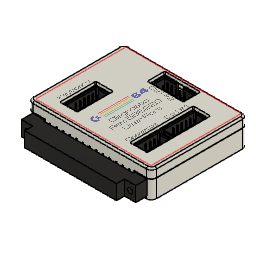
User_Port_Case_wHoles (Autodesk Fusion 360 design; units mm, degrees)
Autodesk Fusion 360 part; units mm, degrees
(part 1 of 2)
sketch "DXF import" plane through (0, 0, 0) normal (0, 0, 1) x (1, 0, 0) in component "PCB"
  arc A0 (0, 1) -> (1, 0) centre (1, 1) ccw
  line L0 (53, 1) -> (53, 54)
  line L1 (0, 1) -> (0, 54)
  arc A1 (53, 54) -> (52, 55) centre (52, 54) ccw
  line L2 (52, 55) -> (1, 55)
  line L3 (1, 0) -> (52, 0)
  arc A2 (1, 55) -> (0, 54) centre (1, 54) ccw
  arc A3 (52, 0) -> (53, 1) centre (52, 1) ccw
  line L4 (39.6875, 41.1163) -> (39.6875, 33.4963)
  line L5 (42.2275, 33.4963) -> (42.2275, 41.1163)
  line L6 (40.9575, 33.4963) -> (40.9575, 32.7343)
  line L7 (40.9575, 41.1163) -> (40.9575, 41.8783)
  line L8 (42.2275, 41.1163) -> (39.6875, 41.1163)
  line L9 (39.6875, 33.4963) -> (42.2275, 33.4963)
  line L10 (15.0813, 41.1163) -> (12.5412, 41.1163)
  line L11 (12.5412, 36.0363) -> (15.0813, 36.0363)
  line L12 (42.4713, 13.38) -> (39.9312, 13.38)
  line L13 (42.4713, 13.38) -> (42.4713, 8.3)
  line L14 (12.5412, 36.0363) -> (12.5412, 41.1163)
  line L15 (15.0813, 41.1163) -> (15.0813, 36.0363)
  line L16 (7.3025, 33.02) -> (12.3825, 33.02)
  line L17 (14.7637, 18.2563) -> (12.2238, 18.2563)
  line L18 (39.9312, 8.3) -> (42.4713, 8.3)
  line L19 (39.9312, 8.3) -> (39.9312, 13.38)
  circle A4 centre (4, 51) radius 3.1
  line L20 (32.6707, 40.7035) -> (32.6707, 34.8615)
  arc A5 (15.9068, 26.1303) -> (15.9068, 28.1623) centre (15.9068, 27.1463) ccw
  line L21 (15.9068, 30.0673) -> (15.9068, 28.1623)
  line L22 (15.9068, 34.8615) -> (32.6707, 34.8615)
  line L23 (15.9068, 24.2253) -> (15.9068, 26.1303)
  line L24 (12.2238, 13.1763) -> (12.2238, 18.2563)
  line L25 (15.9068, 24.2253) -> (32.6707, 24.2253)
  line L26 (32.6707, 30.0673) -> (32.6707, 24.2253)
  line L27 (32.6707, 30.0673) -> (15.9068, 30.0673)
  line L28 (50.18, 0) -> (50.18, -1)
  line L29 (32.6707, 40.7035) -> (15.9068, 40.7035)
  circle A6 centre (49, 51) radius 3.1
  line L30 (15.9068, 18.161) -> (15.9068, 16.256)
  line L31 (46.72, -1) -> (46.72, 0)
  line L32 (12.3825, 30.48) -> (12.3825, 33.02)
  line L33 (15.9068, 12.319) -> (15.9068, 14.224)
  circle A7 centre (49, 51) radius 1.5875
  line L34 (46.72, 0) -> (46.22, 0)
  line L35 (32.6707, 18.161) -> (15.9068, 18.161)
  arc A8 (15.9068, 14.224) -> (15.9068, 16.256) centre (15.9068, 15.24) ccw
  line L36 (15.9068, 12.319) -> (32.6707, 12.319)
  line L37 (32.6707, 18.161) -> (32.6707, 12.319)
  line L38 (49.45, 0.1) -> (49.45, -1)
  line L39 (47.45, 0.1) -> (47.45, -1)
  line L40 (46.22, 0) -> (46.22, -1)
  line L41 (50.68, -1) -> (50.68, 0)
  arc A9 (15.9068, 36.7665) -> (15.9068, 38.7985) centre (15.9068, 37.7825) ccw
  line L42 (50.68, 0) -> (50.18, 0)
  line L43 (31.61, 0.1) -> (31.61, -1)
  line L44 (15.9068, 40.7035) -> (15.9068, 38.7985)
  line L45 (12.2238, 13.1763) -> (14.7637, 13.1763)
  line L46 (14.7637, 18.2563) -> (14.7637, 13.1763)
  line L47 (12.3825, 30.48) -> (7.3025, 30.48)
  line L48 (7.3025, 33.02) -> (7.3025, 30.48)
  circle A10 centre (4, 51) radius 1.5875
  line L49 (15.9068, 34.8615) -> (15.9068, 36.7665)
  line L50 (22.96, 0) -> (22.46, 0)
  line L51 (7.85, 0.1) -> (7.85, -1)
  line L52 (42.76, -1) -> (42.76, 0)
  line L53 (43.49, 0.1) -> (43.49, -1)
  line L54 (45.49, 0.1) -> (45.49, -1)
  line L55 (30.88, -1) -> (30.88, 0)
  line L56 (7.12, -1) -> (7.12, 0)
  line L57 (22.46, 0) -> (22.46, -1)
  line L58 (7.12, 0) -> (6.62, 0)
  line L59 (35.57, 0.1) -> (35.57, -1)
  line L60 (6.62, 0) -> (6.62, -1)
  line L61 (14.54, 0) -> (14.54, -1)
  line L62 (37.57, 0.1) -> (37.57, -1)
  line L63 (38.8, -1) -> (38.8, 0)
  line L64 (15.04, 0) -> (14.54, 0)
  line L65 (18.5, 0) -> (18.5, -1)
  line L66 (29.65, 0.1) -> (29.65, -1)
  line L67 (30.88, 0) -> (30.38, 0)
  line L68 (27.65, 0.1) -> (27.65, -1)
  line L69 (26.42, 0) -> (26.42, -1)
  line L70 (38.8, 0) -> (38.3, 0)
  line L71 (34.84, 0) -> (34.34, 0)
  line L72 (39.53, 0.1) -> (39.53, -1)
  line L73 (42.26, 0) -> (42.26, -1)
  line L74 (42.76, 0) -> (42.26, 0)
  line L75 (26.92, -1) -> (26.92, 0)
  line L76 (38.3, 0) -> (38.3, -1)
  line L77 (33.61, 0.1) -> (33.61, -1)
  line L78 (34.34, 0) -> (34.34, -1)
  line L79 (26.92, 0) -> (26.42, 0)
  line L80 (30.38, 0) -> (30.38, -1)
  line L81 (34.84, -1) -> (34.84, 0)
  line L82 (41.53, 0.1) -> (41.53, -1)
  line L83 (21.73, 0.1) -> (21.73, -1)
  line L84 (15.77, 0.1) -> (15.77, -1)
  line L85 (11.08, -1) -> (11.08, 0)
  line L86 (23.69, 0.1) -> (23.69, -1)
  line L87 (19.73, 0.1) -> (19.73, -1)
  line L88 (25.69, 0.1) -> (25.69, -1)
  line L89 (19, -1) -> (19, 0)
  line L90 (11.81, 0.1) -> (11.81, -1)
  line L91 (54.17, -6.8) -> (54.17, -11.6)
  line L92 (11.08, 0) -> (10.58, 0)
  line L93 (22.96, -1) -> (22.96, 0)
  line L94 (55.97, -6.8) -> (54.17, -6.8)
  line L95 (-6.03, -6.8) -> (-7.58, -6.8)
  line L96 (59.37, -6.8) -> (55.97, -6.8)
  line L97 (60.92, -6.8) -> (59.37, -6.8)
  line L98 (19, 0) -> (18.5, 0)
  line L99 (9.85, 0.1) -> (9.85, -1)
  line L100 (53.47, 0) -> (53.47, -1)
  line L101 (3.16, -1) -> (3.16, 0)
  line L102 (17.77, 0.1) -> (17.77, -1)
  line L103 (-2.63, -6.8) -> (-2.63, -5.2)
  line L104 (-4.33, 0) -> (-4.33, -2.8667)
  line L105 (57.67, -3.6853) -> (57.67, -3.548)
  line L106 (55.97, -4.2) -> (55.97, -2.6)
  line L107 (59.37, -1.6) -> (59.37, 0)
  line L108 (60.92, 0) -> (59.37, 0)
  line L109 (59.37, 0) -> (57.67, 0)
  line L110 (-4.33, -3.548) -> (-4.33, -3.6853)
  line L111 (-4.33, -4.3667) -> (-4.33, -7.2333)
  line L112 (55.97, -1.6) -> (55.97, 0)
  line L113 (57.67, 0) -> (55.97, 0)
  line L114 (-0.83, -6.8) -> (-2.63, -6.8)
  line L115 (-2.63, -4.2) -> (-2.63, -2.6)
  line L116 (-4.33, -8.7333) -> (-4.33, -11.6)
  line L117 (-4.33, 0) -> (-6.03, 0)
  line L118 (10.58, 0) -> (10.58, -1)
  line L119 (13.81, 0.1) -> (13.81, -1)
  line L120 (5.89, 0.1) -> (5.89, -1)
  line L121 (-2.63, -1.6) -> (-2.63, 0)
  line L122 (-6.03, -1.6) -> (-6.03, 0)
  line L123 (55.97, 0) -> (53.47, 0)
  line L124 (-7.58, 0) -> (-7.58, -6.8)
  line L125 (3.16, 0) -> (2.66, 0)
  line L126 (3.89, 0.1) -> (3.89, -1)
  line L127 (15.04, -1) -> (15.04, 0)
  line L128 (59.37, -4.2) -> (59.37, -2.6)
  line L129 (-6.03, -6.8) -> (-6.03, -5.2)
  line L130 (2.66, 0) -> (2.66, -1)
  line L131 (51.81, 14.73) -> (52.6038, 14.73)
  line L132 (52.6038, 23.62) -> (52.6038, 17.27)
  line L133 (-0.13, 0) -> (-2.63, 0)
  line L134 (60.92, 0) -> (60.92, -6.8)
  line L135 (46.2537, 8.38) -> (44.825, 8.38)
  line L136 (51.81, 17.27) -> (52.6038, 17.27)
  line L137 (-0.83, -11.6) -> (-0.83, -6.8)
  line L138 (-6.03, 0) -> (-7.58, 0)
  line L139 (57.67, -2.8667) -> (57.67, 0)
  line L140 (51.3338, 17.27) -> (51.81, 17.27)
  line L141 (46.2537, 23.62) -> (52.6038, 23.62)
  line L142 (44.6662, 22.35) -> (44.825, 22.35)
  line L143 (51.3338, 9.65) -> (46.2537, 9.65)
  line L144 (44.825, 22.35) -> (44.825, 22.8263)
  line L145 (57.67, -11.6) -> (57.67, -8.7333)
  line L146 (43.3962, 23.62) -> (44.825, 23.62)
  line L147 (51.81, 14.73) -> (51.81, 9.1737)
  line L148 (46.2537, 22.35) -> (46.2537, 22.8263)
  line L149 (57.67, -7.2333) -> (57.67, -4.3667)
  line L150 (44.825, 8.38) -> (43.3962, 8.38)
  line L151 (51.3338, 22.35) -> (51.3338, 17.27)
  line L152 (44.825, 9.65) -> (44.825, 9.1737)
  line L153 (55.97, -6.8) -> (55.97, -5.2)
  line L154 (51.3338, 22.35) -> (51.81, 22.8263)
  line L155 (51.3338, 14.73) -> (51.3338, 9.65)
  line L156 (-4.33, -7.9147) -> (-4.33, -8.052)
  line L157 (53.47, -1) -> (-0.13, -1)
  line L158 (-2.63, -6.8) -> (-6.03, -6.8)
  line L159 (44.6662, 9.65) -> (44.6662, 22.35)
  line L160 (46.2537, 22.35) -> (51.3338, 22.35)
  line L161 (54.17, -11.6) -> (-0.83, -11.6)
  line L162 (57.67, -8.052) -> (57.67, -7.9147)
  line L163 (52.6038, 14.73) -> (52.6038, 8.38)
  line L164 (51.3338, 17.27) -> (51.3338, 14.73)
  line L165 (43.3962, 8.38) -> (43.3962, 23.62)
  line L166 (46.2537, 9.65) -> (44.825, 9.65)
  line L167 (51.3338, 14.73) -> (51.81, 14.73)
  line L168 (-6.03, -4.2) -> (-6.03, -2.6)
  line L169 (52.6038, 17.27) -> (52.6038, 14.73)
  line L170 (52.6038, 8.38) -> (46.2537, 8.38)
  line L171 (44.825, 9.65) -> (44.6662, 9.65)
  line L172 (59.37, -6.8) -> (59.37, -5.2)
  line L173 (44.825, 23.62) -> (46.2537, 23.62)
  line L174 (44.825, 22.35) -> (46.2537, 22.35)
  line L175 (-2.63, 0) -> (-4.33, 0)
  line L176 (-0.13, -1) -> (-0.13, 0)
  arc A11 (43.3962, 35.4763) -> (43.3962, 34.3651) centre (43.3962, 34.9207) ccw
  line L177 (46.2537, 9.1737) -> (51.81, 9.1737)
  line L178 (44.19, 9.1737) -> (44.6662, 9.65)
  arc A12 (43.3962, 10.92) -> (43.3962, 9.65) centre (43.3962, 10.285) ccw
  line L179 (44.825, 22.8263) -> (44.19, 22.8263)
  arc A13 (43.3962, 27.38) -> (43.3962, 26.11) centre (43.3962, 26.745) ccw
  line L180 (44.825, 24.84) -> (43.3962, 24.84)
  line L181 (44.825, 25.6337) -> (44.825, 24.84)
  line L182 (51.81, 25.6337) -> (51.3338, 26.11)
  arc A14 (43.3962, 22.35) -> (43.3962, 21.08) centre (43.3962, 21.715) ccw
  line L183 (44.19, 25.6337) -> (44.825, 25.6337)
  line L184 (44.6662, 26.11) -> (44.6662, 43.89)
  line L185 (44.825, 26.11) -> (44.6662, 26.11)
  line L186 (43.3962, 45.16) -> (44.825, 45.16)
  line L187 (46.2537, 44.3663) -> (46.2537, 45.16)
  line L188 (44.825, 43.89) -> (44.825, 44.3663)
  line L189 (51.81, 9.1737) -> (51.3338, 9.65)
  arc A15 (43.3962, 16.4763) -> (43.3962, 15.3651) centre (43.3962, 15.9207) ccw
  line L190 (46.2537, 22.8263) -> (46.2537, 23.62)
  line L191 (44.19, 9.1737) -> (44.825, 9.1737)
  line L192 (44.825, 9.1737) -> (44.825, 8.38)
  line L193 (51.81, 17.27) -> (51.81, 22.8263)
  line L194 (46.2537, 9.65) -> (46.2537, 9.1737)
  line L195 (46.2537, 22.8263) -> (51.81, 22.8263)
  line L196 (44.6662, 22.35) -> (44.19, 22.8263)
  line L197 (51.3338, 37.0638) -> (51.3338, 32.9362)
  line L198 (51.3338, 37.0638) -> (51.81, 37.0638)
  line L199 (44.825, 44.3663) -> (44.19, 44.3663)
  line L200 (51.3338, 43.89) -> (51.81, 44.3663)
  line L201 (44.825, 43.89) -> (46.2537, 43.89)
  line L202 (46.2537, 25.6337) -> (46.2537, 24.84)
  line L203 (51.3338, 43.89) -> (51.3338, 37.0638)
  line L204 (46.2537, 43.89) -> (46.2537, 44.3663)
  line L205 (51.81, 32.9362) -> (52.6038, 32.9362)
  line L206 (51.3338, 26.11) -> (46.2537, 26.11)
  line L207 (46.2537, 9.1737) -> (46.2537, 8.38)
  line L208 (44.19, 25.6337) -> (44.19, 44.3663)
  line L209 (44.19, 9.1737) -> (44.19, 22.8263)
  line L210 (46.2537, 25.6337) -> (51.81, 25.6337)
  line L211 (44.19, 25.6337) -> (44.6662, 26.11)
  line L212 (44.825, 22.8263) -> (44.825, 23.62)
  line L213 (51.81, 32.9362) -> (51.81, 25.6337)
  line L214 (44.6662, 43.89) -> (44.825, 43.89)
  arc A16 (43.3962, 43.89) -> (43.3962, 42.62) centre (43.3962, 43.255) ccw
  line L215 (44.825, 26.11) -> (44.825, 25.6337)
  line L216 (52.6038, 37.0638) -> (52.6038, 32.9362)
  line L217 (43.3962, 24.84) -> (43.3962, 45.16)
  line L218 (46.2537, 26.11) -> (44.825, 26.11)
  line L219 (44.825, 44.3663) -> (44.825, 45.16)
  line L220 (37.16, 46.825) -> (37.16, 45.3962)
  line L221 (18.11, 48.2537) -> (17.6337, 48.2537)
  line L222 (37.16, 54.6038) -> (37.16, 48.2537)
  arc A17 (26.5238, 45.3962) -> (27.635, 45.3962) centre (27.0794, 45.3962) ccw
  line L223 (51.3338, 32.9362) -> (51.3338, 26.11)
  line L224 (36.3663, 46.19) -> (36.3663, 46.825)
  line L225 (51.81, 37.0638) -> (51.81, 44.3663)
  line L226 (29.0638, 53.81) -> (29.0638, 54.6038)
  line L227 (29.0638, 53.3338) -> (35.89, 53.3338)
  line L228 (46.2537, 45.16) -> (52.6038, 45.16)
  line L229 (17.6337, 46.825) -> (16.84, 46.825)
  line L230 (37.16, 48.2537) -> (37.16, 46.825)
  line L231 (46.2537, 43.89) -> (51.3338, 43.89)
  line L232 (52.6038, 32.9362) -> (52.6038, 24.84)
  line L233 (18.11, 53.3338) -> (24.9362, 53.3338)
  line L234 (36.3663, 48.2537) -> (36.3663, 53.81)
  line L235 (52.6038, 45.16) -> (52.6038, 37.0638)
  line L236 (51.3338, 32.9362) -> (51.81, 32.9362)
  line L237 (44.6662, 43.89) -> (44.19, 44.3663)
  line L238 (17.6337, 46.825) -> (17.6337, 46.19)
  line L239 (18.11, 46.6662) -> (18.11, 46.825)
  line L240 (52.6038, 24.84) -> (46.2537, 24.84)
  line L241 (18.11, 46.825) -> (18.11, 48.2537)
  line L242 (24.9362, 53.81) -> (24.9362, 54.6038)
  line L243 (29.0638, 54.6038) -> (37.16, 54.6038)
  line L244 (29.0638, 53.3338) -> (29.0638, 53.81)
  line L245 (18.11, 46.825) -> (17.6337, 46.825)
  line L246 (36.3663, 46.19) -> (17.6337, 46.19)
  line L247 (46.2537, 44.3663) -> (51.81, 44.3663)
  line L248 (29.0638, 53.81) -> (36.3663, 53.81)
  line L249 (18.11, 53.3338) -> (17.6337, 53.81)
  line L250 (44.825, 45.16) -> (46.2537, 45.16)
  line L251 (46.2537, 24.84) -> (44.825, 24.84)
  arc A18 (18.11, 45.3962) -> (19.38, 45.3962) centre (18.745, 45.3962) ccw
  line L252 (24.9362, 53.3338) -> (29.0638, 53.3338)
  line L253 (46.2537, 26.11) -> (46.2537, 25.6337)
  line L254 (18.11, 46.6662) -> (17.6337, 46.19)
  line L255 (36.3663, 46.19) -> (35.89, 46.6662)
  line L256 (51.81, 37.0638) -> (52.6038, 37.0638)
  line L257 (35.89, 48.2537) -> (35.89, 46.825)
  line L258 (2.6987, 27.4638) -> (2.8575, 27.4638)
  line L259 (16.84, 46.825) -> (16.84, 48.2537)
  line L260 (9.3663, 9.6837) -> (4.2862, 9.6837)
  line L261 (9.8425, 20.6376) -> (9.8425, 27.9401)
  line L262 (18.11, 48.2537) -> (18.11, 53.3338)
  line L263 (4.2862, 28.7338) -> (10.6363, 28.7338)
  line L264 (9.3663, 16.5099) -> (9.3663, 9.6837)
  arc A19 (1.4287, 27.4638) -> (1.4287, 26.1938) centre (1.4287, 26.8288) ccw
  line L265 (10.6363, 28.7338) -> (10.6363, 20.6376)
  line L266 (2.8575, 9.6837) -> (2.6987, 9.6837)
  line L267 (24.9362, 53.3338) -> (24.9362, 53.81)
  arc A20 (34.62, 45.3962) -> (35.89, 45.3962) centre (35.255, 45.3962) ccw
  line L268 (9.3663, 20.6376) -> (9.3663, 16.5099)
  line L269 (17.6337, 48.2537) -> (16.84, 48.2537)
  line L270 (24.9362, 53.81) -> (17.6337, 53.81)
  line L271 (2.6987, 27.4638) -> (2.2225, 27.9401)
  line L272 (4.2862, 9.6837) -> (4.2862, 9.2074)
  line L273 (36.3663, 46.825) -> (37.16, 46.825)
  line L274 (16.84, 54.6038) -> (24.9362, 54.6038)
  line L275 (35.89, 48.2537) -> (36.3663, 48.2537)
  line L276 (17.6337, 48.2537) -> (17.6337, 53.81)
  line L277 (16.84, 45.3962) -> (16.84, 46.825)
  line L278 (35.89, 53.3338) -> (35.89, 48.2537)
  line L279 (10.6363, 20.6376) -> (10.6363, 16.5099)
  line L280 (2.8575, 28.7338) -> (4.2862, 28.7338)
  line L281 (35.89, 46.6662) -> (18.11, 46.6662)
  line L282 (24.9362, 54.6038) -> (29.0638, 54.6038)
  line L283 (1.4287, 28.7338) -> (2.8575, 28.7338)
  line L284 (35.89, 46.825) -> (36.3663, 46.825)
  line L285 (36.3663, 48.2537) -> (37.16, 48.2537)
  line L286 (35.89, 46.825) -> (35.89, 46.6662)
  line L287 (2.8575, 8.4138) -> (1.4287, 8.4138)
  line L288 (1.4287, 8.4138) -> (1.4287, 28.7338)
  line L289 (37.16, 45.3962) -> (16.84, 45.3962)
  line L290 (10.6363, 16.5099) -> (10.6363, 8.4138)
  line L291 (4.2862, 27.9401) -> (4.2862, 28.7338)
  arc A21 (1.4287, 10.9537) -> (1.4287, 9.6837) centre (1.4287, 10.3187) ccw
  line L292 (9.3663, 20.6376) -> (9.8425, 20.6376)
  line L293 (36.3663, 53.81) -> (35.89, 53.3338)
  line L294 (2.8575, 27.9401) -> (2.2225, 27.9401)
  line L295 (9.3663, 16.5099) -> (9.8425, 16.5099)
  line L296 (2.8575, 9.6837) -> (2.8575, 9.2074)
  line L297 (2.2225, 9.2074) -> (2.6987, 9.6837)
  arc A22 (1.4287, 19.05) -> (1.4287, 17.9388) centre (1.4287, 18.4944) ccw
  line L298 (16.84, 48.2537) -> (16.84, 54.6038)
  line L299 (4.2862, 27.4638) -> (9.3663, 27.4638)
  line L300 (36.6713, 26.035) -> (34.1313, 26.035)
  line L301 (38.1, 33.4963) -> (38.1, 32.7343)
  line L302 (36.9888, 26.035) -> (36.9888, 18.415)
  line L303 (4.2862, 9.2074) -> (9.8425, 9.2074)
  line L304 (39.37, 33.4963) -> (39.37, 41.1163)
  line L305 (2.8575, 9.2074) -> (2.8575, 8.4138)
  line L306 (39.5288, 26.035) -> (36.9888, 26.035)
  line L307 (38.2587, 18.415) -> (38.2587, 17.653)
  line L308 (36.9888, 18.415) -> (39.5288, 18.415)
  line L309 (36.6713, 18.415) -> (36.6713, 26.035)
  line L310 (9.8425, 16.5099) -> (9.8425, 9.2074)
  line L311 (10.6363, 8.4138) -> (4.2862, 8.4138)
  line L312 (34.1313, 18.415) -> (36.6713, 18.415)
  line L313 (9.8425, 20.6376) -> (10.6363, 20.6376)
  line L314 (9.3663, 27.4638) -> (9.3663, 20.6376)
  line L315 (2.2225, 9.2074) -> (2.2225, 27.9401)
  line L316 (2.8575, 27.4638) -> (4.2862, 27.4638)
  line L317 (2.8575, 27.4638) -> (2.8575, 27.9401)
  line L318 (34.1313, 26.035) -> (34.1313, 18.415)
  line L319 (39.5288, 18.415) -> (39.5288, 26.035)
  line L320 (36.83, 33.4963) -> (39.37, 33.4963)
  line L321 (2.6987, 9.6837) -> (2.6987, 27.4638)
  line L322 (2.2225, 9.2074) -> (2.8575, 9.2074)
  line L323 (9.8425, 9.2074) -> (9.3663, 9.6837)
  line L324 (35.4013, 18.415) -> (35.4013, 17.653)
  line L325 (9.8425, 16.5099) -> (10.6363, 16.5099)
  line L326 (38.1, 41.1163) -> (38.1, 41.8783)
  line L327 (35.4013, 26.035) -> (35.4013, 26.797)
  line L328 (4.2862, 8.4138) -> (2.8575, 8.4138)
  line L329 (36.83, 41.1163) -> (36.83, 33.4963)
  line L330 (2.8575, 27.9401) -> (2.8575, 28.7338)
  line L331 (4.2862, 9.2074) -> (4.2862, 8.4138)
  line L332 (39.37, 41.1163) -> (36.83, 41.1163)
  line L333 (4.2862, 27.9401) -> (9.8425, 27.9401)
  line L334 (9.3663, 27.4638) -> (9.8425, 27.9401)
  line L335 (4.2862, 27.4638) -> (4.2862, 27.9401)
  line L336 (4.2862, 9.6837) -> (2.8575, 9.6837)
  line L337 (11.5888, 43.6088) -> (11.5888, 42.8468)
  line L338 (39.8463, 26.035) -> (39.8463, 18.415)
  line L339 (10.3187, 51.2288) -> (10.3187, 43.6088)
  line L340 (15.0813, 22.86) -> (15.0813, 30.48)
  line L341 (13.335, 51.2288) -> (13.335, 43.6088)
  line L342 (13.8113, 22.86) -> (13.8113, 22.098)
  line L343 (38.2587, 26.035) -> (38.2587, 26.797)
  line L344 (42.3863, 26.035) -> (39.8463, 26.035)
  line L345 (15.875, 51.2288) -> (13.335, 51.2288)
  line L346 (13.335, 43.6088) -> (15.875, 43.6088)
  line L347 (42.3863, 18.415) -> (42.3863, 26.035)
  line L348 (14.605, 51.2288) -> (14.605, 51.9908)
  line L349 (13.8113, 30.48) -> (13.8113, 31.242)
  line L350 (12.5412, 30.48) -> (12.5412, 22.86)
  line L351 (12.8588, 43.6088) -> (12.8588, 51.2288)
  line L352 (15.0813, 30.48) -> (12.5412, 30.48)
  line L353 (11.5888, 51.2288) -> (11.5888, 51.9908)
  line L354 (12.8588, 51.2288) -> (10.3187, 51.2288)
  line L355 (10.3187, 43.6088) -> (12.8588, 43.6088)
  line L356 (41.1163, 26.035) -> (41.1163, 26.797)
  line L357 (15.875, 43.6088) -> (15.875, 51.2288)
  line L358 (12.5412, 22.86) -> (15.0813, 22.86)
  line L359 (41.1163, 18.415) -> (41.1163, 17.653)
  line L360 (14.605, 43.6088) -> (14.605, 42.8468)
  line L361 (39.8463, 18.415) -> (42.3863, 18.415)
  line L362 (52, 0) -> (59.45, 0)
  line L363 (27.254, 51.016) -> (27.254, 51.524)
  line L364 (24.206, 48.476) -> (24.714, 48.476)
  line L365 (26.746, 48.984) -> (26.746, 48.476)
  line L366 (32.334, 48.984) -> (31.826, 48.984)
  line L367 (32.334, 51.524) -> (31.826, 51.524)
  line L368 (26.746, 48.476) -> (27.254, 48.476)
  line L369 (24.714, 51.016) -> (24.714, 51.524)
  line L370 (21.666, 48.984) -> (21.666, 48.476)
  line L371 (21.666, 48.476) -> (22.174, 48.476)
  line L372 (31.826, 48.476) -> (32.334, 48.476)
  line L373 (24.714, 48.476) -> (24.714, 48.984)
  line L374 (21.666, 51.524) -> (21.666, 51.016)
  line L375 (27.254, 48.476) -> (27.254, 48.984)
  line L376 (24.206, 51.016) -> (24.714, 51.016)
  line L377 (29.794, 51.524) -> (29.286, 51.524)
  line L378 (21.666, 51.016) -> (22.174, 51.016)
  line L379 (24.206, 48.984) -> (24.206, 48.476)
  line L380 (27.254, 51.524) -> (26.746, 51.524)
  line L381 (29.286, 51.524) -> (29.286, 51.016)
  line L382 (22.174, 48.984) -> (21.666, 48.984)
  line L383 (31.826, 51.524) -> (31.826, 51.016)
  line L384 (29.286, 48.984) -> (29.286, 48.476)
  line L385 (29.286, 51.016) -> (29.794, 51.016)
  line L386 (26.746, 51.524) -> (26.746, 51.016)
  line L387 (32.334, 48.476) -> (32.334, 48.984)
  line L388 (22.174, 51.524) -> (21.666, 51.524)
  line L389 (29.794, 48.476) -> (29.794, 48.984)
  line L390 (49.016, 32.206) -> (49.524, 32.206)
  line L391 (31.826, 51.016) -> (32.334, 51.016)
  line L392 (24.206, 51.524) -> (24.206, 51.016)
  line L393 (29.794, 51.016) -> (29.794, 51.524)
  line L394 (31.826, 48.984) -> (31.826, 48.476)
  line L395 (22.174, 51.016) -> (22.174, 51.524)
  line L396 (32.334, 51.016) -> (32.334, 51.524)
  line L397 (29.286, 48.476) -> (29.794, 48.476)
  line L398 (27.254, 48.984) -> (26.746, 48.984)
  line L399 (22.174, 48.476) -> (22.174, 48.984)
  line L400 (24.714, 51.524) -> (24.206, 51.524)
  line L401 (26.746, 51.016) -> (27.254, 51.016)
  line L402 (24.714, 48.984) -> (24.206, 48.984)
  line L403 (29.794, 48.984) -> (29.286, 48.984)
  line L404 (5.0165, 15.7798) -> (5.0165, 16.2878)
  line L405 (7.5565, 16.2878) -> (7.0485, 16.2878)
  line L406 (7.5565, 20.8597) -> (7.5565, 21.3677)
  line L407 (7.0485, 18.8278) -> (7.0485, 18.3198)
  line L408 (5.0165, 23.3998) -> (5.0165, 23.9078)
  line L409 (5.0165, 13.7478) -> (4.5085, 13.7478)
  line L410 (7.0485, 20.8597) -> (7.5565, 20.8597)
  line L411 (7.0485, 13.2398) -> (7.5565, 13.2398)
  line L412 (5.0165, 20.8597) -> (5.0165, 21.3677)
  line L413 (5.0165, 18.3198) -> (5.0165, 18.8278)
  line L414 (4.5085, 15.7798) -> (5.0165, 15.7798)
  line L415 (5.0165, 16.2878) -> (4.5085, 16.2878)
  line L416 (5.0165, 13.2398) -> (5.0165, 13.7478)
  line L417 (5.0165, 18.8278) -> (4.5085, 18.8278)
  line L418 (7.0485, 16.2878) -> (7.0485, 15.7798)
  line L419 (7.5565, 18.3198) -> (7.5565, 18.8278)
  line L420 (4.5085, 18.8278) -> (4.5085, 18.3198)
  line L421 (7.5565, 13.7478) -> (7.0485, 13.7478)
  line L422 (7.0485, 21.3677) -> (7.0485, 20.8597)
  line L423 (7.0485, 18.3198) -> (7.5565, 18.3198)
  line L424 (4.5085, 16.2878) -> (4.5085, 15.7798)
  line L425 (4.5085, 13.7478) -> (4.5085, 13.2398)
  line L426 (7.0485, 15.7798) -> (7.5565, 15.7798)
  line L427 (4.5085, 18.3198) -> (5.0165, 18.3198)
  line L428 (7.5565, 15.7798) -> (7.5565, 16.2878)
  line L429 (7.5565, 18.8278) -> (7.0485, 18.8278)
  line L430 (4.5085, 20.8597) -> (5.0165, 20.8597)
  line L431 (7.5565, 13.2398) -> (7.5565, 13.7478)
  line L432 (7.5565, 21.3677) -> (7.0485, 21.3677)
  line L433 (7.0485, 13.7478) -> (7.0485, 13.2398)
  line L434 (4.5085, 21.3677) -> (4.5085, 20.8597)
  line L435 (7.0485, 23.3998) -> (7.5565, 23.3998)
  line L436 (45.49, 0.1) -> (45.49, 4)
  line L437 (49.45, 0.1) -> (49.45, 4)
  line L438 (47.95, 3) -> (47.95, 2)
  line L439 (35.57, 0.1) -> (35.57, 4)
  line L440 (7.5565, 23.9078) -> (7.0485, 23.9078)
  line L441 (48.95, 3) -> (48.95, 2)
  line L442 (4.5085, 13.2398) -> (5.0165, 13.2398)
  line L443 (7.5565, 23.3998) -> (7.5565, 23.9078)
  arc A23 (49.45, 4) -> (47.45, 4) centre (48.45, 4) ccw
  line L444 (47.45, 0.1) -> (47.45, 4)
  line L445 (5.0165, 21.3677) -> (4.5085, 21.3677)
  arc A24 (48.95, 3) -> (47.95, 3) centre (48.45, 3) ccw
  arc A25 (47.95, 2) -> (48.95, 2) centre (48.45, 2) ccw
  line L446 (4.5085, 23.9078) -> (4.5085, 23.3998)
  line L447 (7.0485, 23.9078) -> (7.0485, 23.3998)
  line L448 (5.0165, 23.9078) -> (4.5085, 23.9078)
  line L449 (4.5085, 23.3998) -> (5.0165, 23.3998)
  arc A26 (29.15, 3) -> (28.15, 3) centre (28.65, 3) ccw
  arc A27 (25.69, 4) -> (23.69, 4) centre (24.69, 4) ccw
  line L450 (37.07, 3) -> (37.07, 2)
  arc A28 (43.99, 2) -> (44.99, 2) centre (44.49, 2) ccw
  line L451 (43.99, 3) -> (43.99, 2)
  line L452 (32.11, 3) -> (32.11, 2)
  arc A29 (44.99, 3) -> (43.99, 3) centre (44.49, 3) ccw
  line L453 (43.49, 0.1) -> (43.49, 4)
  arc A30 (37.07, 3) -> (36.07, 3) centre (36.57, 3) ccw
  arc A31 (40.03, 2) -> (41.03, 2) centre (40.53, 2) ccw
  arc A32 (33.61, 4) -> (31.61, 4) centre (32.61, 4) ccw
  line L454 (40.03, 3) -> (40.03, 2)
  line L455 (25.69, 0.1) -> (25.69, 4)
  arc A33 (28.15, 2) -> (29.15, 2) centre (28.65, 2) ccw
  line L456 (31.61, 0.1) -> (31.61, 4)
  arc A34 (45.49, 4) -> (43.49, 4) centre (44.49, 4) ccw
  line L457 (29.15, 3) -> (29.15, 2)
  arc A35 (25.19, 3) -> (24.19, 3) centre (24.69, 3) ccw
  line L458 (44.99, 3) -> (44.99, 2)
  arc A36 (41.03, 3) -> (40.03, 3) centre (40.53, 3) ccw
  arc A37 (41.53, 4) -> (39.53, 4) centre (40.53, 4) ccw
  line L459 (23.69, 0.1) -> (23.69, 4)
  line L460 (36.07, 3) -> (36.07, 2)
  line L461 (37.57, 0.1) -> (37.57, 4)
  line L462 (41.03, 3) -> (41.03, 2)
  line L463 (27.65, 0.1) -> (27.65, 4)
  line L464 (25.19, 3) -> (25.19, 2)
  line L465 (28.15, 3) -> (28.15, 2)
  line L466 (29.65, 0.1) -> (29.65, 4)
  line L467 (33.61, 0.1) -> (33.61, 4)
  arc A38 (13.81, 4) -> (11.81, 4) centre (12.81, 4) ccw
  line L468 (5.89, 0.1) -> (5.89, 4)
  line L469 (21.23, 3) -> (21.23, 2)
  line L470 (8.35, 3) -> (8.35, 2)
  line L471 (21.73, 0.1) -> (21.73, 4)
  line L472 (9.85, 0.1) -> (9.85, 4)
  line L473 (13.81, 0.1) -> (13.81, 4)
  line L474 (13.31, 3) -> (13.31, 2)
  arc A39 (12.31, 2) -> (13.31, 2) centre (12.81, 2) ccw
  line L475 (3.89, 0.1) -> (3.89, 4)
  line L476 (4.39, 3) -> (4.39, 2)
  arc A40 (29.65, 4) -> (27.65, 4) centre (28.65, 4) ccw
  arc A41 (37.57, 4) -> (35.57, 4) centre (36.57, 4) ccw
  line L477 (19.73, 0.1) -> (19.73, 4)
  arc A42 (9.35, 3) -> (8.35, 3) centre (8.85, 3) ccw
  line L478 (41.53, 0.1) -> (41.53, 4)
  line L479 (11.81, 0.1) -> (11.81, 4)
  arc A43 (36.07, 2) -> (37.07, 2) centre (36.57, 2) ccw
  arc A44 (17.27, 3) -> (16.27, 3) centre (16.77, 3) ccw
  line L480 (33.11, 3) -> (33.11, 2)
  line L481 (15.77, 0.1) -> (15.77, 4)
  line L482 (20.23, 3) -> (20.23, 2)
  line L483 (17.27, 3) -> (17.27, 2)
  line L484 (9.35, 3) -> (9.35, 2)
  arc A45 (13.31, 3) -> (12.31, 3) centre (12.81, 3) ccw
  line L485 (17.77, 0.1) -> (17.77, 4)
  arc A46 (5.39, 3) -> (4.39, 3) centre (4.89, 3) ccw
  line L486 (12.31, 3) -> (12.31, 2)
  arc A47 (8.35, 2) -> (9.35, 2) centre (8.85, 2) ccw
  line L487 (5.39, 3) -> (5.39, 2)
  arc A48 (32.11, 2) -> (33.11, 2) centre (32.61, 2) ccw
  arc A49 (33.11, 3) -> (32.11, 3) centre (32.61, 3) ccw
  line L488 (39.53, 0.1) -> (39.53, 4)
  arc A50 (24.19, 2) -> (25.19, 2) centre (24.69, 2) ccw
  arc A51 (9.85, 4) -> (7.85, 4) centre (8.85, 4) ccw
  arc A52 (21.23, 3) -> (20.23, 3) centre (20.73, 3) ccw
  line L489 (49.524, 16.254) -> (49.016, 16.254)
  line L490 (46.984, 16.254) -> (46.476, 16.254)
  line L491 (49.016, 15.746) -> (49.524, 15.746)
  arc A53 (5.89, 4) -> (3.89, 4) centre (4.89, 4) ccw
  line L492 (46.984, 18.794) -> (46.476, 18.794)
  arc A54 (4.39, 2) -> (5.39, 2) centre (4.89, 2) ccw
  line L493 (46.476, 16.254) -> (46.476, 15.746)
  line L494 (49.016, 13.714) -> (49.016, 13.206)
  line L495 (7.85, 0.1) -> (7.85, 4)
  line L496 (49.524, 15.746) -> (49.524, 16.254)
  line L497 (49.524, 13.714) -> (49.016, 13.714)
  line L498 (16.27, 3) -> (16.27, 2)
  line L499 (46.984, 13.206) -> (46.984, 13.714)
  line L500 (24.19, 3) -> (24.19, 2)
  arc A55 (21.73, 4) -> (19.73, 4) centre (20.73, 4) ccw
  line L501 (46.476, 13.206) -> (46.984, 13.206)
  arc A56 (16.27, 2) -> (17.27, 2) centre (16.77, 2) ccw
  line L502 (46.476, 18.794) -> (46.476, 18.286)
  arc A57 (17.77, 4) -> (15.77, 4) centre (16.77, 4) ccw
  line L503 (46.984, 18.286) -> (46.984, 18.794)
  line L504 (46.476, 15.746) -> (46.984, 15.746)
  arc A58 (20.23, 2) -> (21.23, 2) centre (20.73, 2) ccw
  line L505 (46.984, 15.746) -> (46.984, 16.254)
  line L506 (49.016, 39.826) -> (49.524, 39.826)
  line L507 (49.524, 32.714) -> (49.016, 32.714)
  line L508 (46.984, 35.254) -> (46.476, 35.254)
  line L509 (49.524, 40.334) -> (49.016, 40.334)
  line L510 (46.476, 32.714) -> (46.476, 32.206)
  line L511 (46.476, 35.254) -> (46.476, 34.746)
  line L512 (49.016, 30.174) -> (49.016, 29.666)
  line L513 (49.016, 37.286) -> (49.524, 37.286)
  line L514 (46.476, 18.286) -> (46.984, 18.286)
  line L515 (49.016, 32.714) -> (49.016, 32.206)
  line L516 (46.476, 34.746) -> (46.984, 34.746)
  line L517 (46.476, 32.206) -> (46.984, 32.206)
  line L518 (49.524, 37.286) -> (49.524, 37.794)
  line L519 (46.984, 13.714) -> (46.476, 13.714)
  line L520 (49.016, 13.206) -> (49.524, 13.206)
  line L521 (46.476, 29.666) -> (46.984, 29.666)
  line L522 (49.016, 37.794) -> (49.016, 37.286)
  line L523 (49.524, 30.174) -> (49.016, 30.174)
  line L524 (49.016, 29.666) -> (49.524, 29.666)
  line L525 (49.524, 32.206) -> (49.524, 32.714)
  line L526 (46.476, 30.174) -> (46.476, 29.666)
  line L527 (46.984, 34.746) -> (46.984, 35.254)
  line L528 (46.476, 40.334) -> (46.476, 39.826)
  line L529 (46.476, 37.286) -> (46.984, 37.286)
  line L530 (49.016, 34.746) -> (49.524, 34.746)
  line L531 (46.476, 37.794) -> (46.476, 37.286)
  line L532 (46.984, 39.826) -> (46.984, 40.334)
  line L533 (46.984, 37.794) -> (46.476, 37.794)
  line L534 (49.524, 18.286) -> (49.524, 18.794)
  line L535 (49.524, 13.206) -> (49.524, 13.714)
  line L536 (49.016, 18.286) -> (49.524, 18.286)
  line L537 (49.524, 18.794) -> (49.016, 18.794)
  line L538 (49.016, 35.254) -> (49.016, 34.746)
  line L539 (46.476, 39.826) -> (46.984, 39.826)
  line L540 (46.984, 32.714) -> (46.476, 32.714)
  line L541 (49.524, 37.794) -> (49.016, 37.794)
  line L542 (46.476, 13.714) -> (46.476, 13.206)
  line L543 (49.524, 39.826) -> (49.524, 40.334)
  line L544 (46.984, 37.286) -> (46.984, 37.794)
  line L545 (49.524, 29.666) -> (49.524, 30.174)
  line L546 (49.016, 18.794) -> (49.016, 18.286)
  line L547 (49.016, 40.334) -> (49.016, 39.826)
  line L548 (46.984, 29.666) -> (46.984, 30.174)
  line L549 (46.984, 40.334) -> (46.476, 40.334)
  line L550 (49.016, 16.254) -> (49.016, 15.746)
  line L551 (46.984, 30.174) -> (46.476, 30.174)
  line L552 (49.524, 35.254) -> (49.016, 35.254)
  line L553 (49.524, 34.746) -> (49.524, 35.254)
  line L554 (46.984, 32.206) -> (46.984, 32.714)
extrude "Extrude1" add sketch "DXF import" against normal blind 1.6 contours A0 L0 L1 A1 L2 L3 A2 A3 L34 L38 L39 L42 L43 L50 L51 L53 L54 L58 L59 L62 L64 L66 L67 L68 L70 L71 L72 L74 L77 L79 L82 L83 L84 L86 L87 L88 L90 L92 L98 L99 L102 L119 L120 L125 L126 L436 L437 L439 A23 L444 A27 L453 A32 L455 L456 A34 A37 L459 L461 L463 L466 L467 A38 L468 L471 L472 L473 L475 A40 A41 L477 L478 L479 L481 L485 L488 A51 A53 L495 A55 A57 | L3 L120 L126 L468 L475 A53 | L3 L51 L99 L472 A51 L495 | L3 L38 L39 L437 A23 L444 | L3 L90 L119 A38 L473 L479 | L3 L53 L54 L436 L453 A34 | L3 L84 L102 L481 L485 A57 | L3 L72 L82 A37 L478 L488 | L3 L83 L87 L471 L477 A55 | L3 L59 L62 L439 L461 A41 | L3 L86 L88 A27 L455 L459 | L3 L43 L77 A32 L456 L467 | L3 L66 L68 L463 L466 A40 | L4 L5 L8 L9 | L10 L11 L14 L15 | L12 L13 L18 L19 | L16 L32 L47 L48 | L17 L24 L45 L46 | A4 | L20 L22 L29 A9 L44 L49 | A5 L21 L23 L25 L26 L27 | A6 | L30 L33 L35 A8 L36 L37 | L131 L136 L140 L164 L167 L169 | L131 L147 L163 L170 L177 L207 | L147 L155 L167 L189 | L143 L177 L189 L194 | L142 L143 L151 L155 L159 L160 L164 L166 L171 L174 | L132 L136 L141 L190 L193 L195 | L135 L152 L166 L192 L194 L207 | L140 L151 L154 L193 | L148 L154 L160 L195 | L146 L150 L165 L179 L191 L192 L209 L212 | L144 L148 L173 L174 L190 L212 | L152 L171 L178 L191 | L159 L178 L196 L209 | L142 L144 L179 L196 | L165 A12 | L165 A14 | L165 A15 | A11 L217 | L180 L181 L183 L186 L199 L208 L217 L219 | A16 L217 | A13 L217 | L187 L188 L201 L204 L219 L250 | L181 L202 L215 L218 L251 L253 | L188 L199 L214 L237 | L187 L225 L228 L235 L247 L256 | L183 L185 L211 L215 | L202 L205 L210 L213 L232 L240 | L184 L185 L197 L201 L203 L206 L214 L218 L223 L231 | L184 L208 L211 L237 | L200 L204 L231 L247 | L182 L206 L210 L253 | L198 L200 L203 L225 | L197 L198 L205 L216 L236 L256 | L182 L213 L223 L236 | L230 L257 L273 L275 L284 L285 | L220 L224 L229 L238 L246 L273 L277 L289 | L222 L226 L234 L243 L248 L285 | L224 L255 L284 L286 | A20 L289 | L234 L275 L278 L293 | L246 L254 L255 L281 | L227 L233 L239 L241 L252 L257 L262 L278 L281 L286 | L226 L242 L244 L252 L267 L282 | L227 L244 L248 L293 | L238 L239 L245 L254 | A17 L289 | L242 L269 L270 L274 L276 L298 | L221 L229 L241 L245 L259 L269 | L233 L249 L267 L270 | A18 L289 | L221 L249 L262 L276 | L258 L271 L294 L317 | L271 L297 L315 L321 | L258 L260 L264 L266 L268 L299 L314 L316 L321 L336 | L280 L291 L316 L317 L330 L335 | L283 L287 L288 L294 L305 L315 L322 L330 | L266 L296 L297 L322 | L299 L333 L334 L335 | L272 L296 L305 L328 L331 L336 | L261 L292 L314 L334 | L261 L263 L265 L291 L313 L333 | L260 L272 L303 L323 | L268 L279 L292 L295 L313 L325 | L264 L295 L310 L323 | L290 L303 L310 L311 L325 L331 | A19 L288 | L288 A21 | L288 A22 | L300 L309 L312 L318 | L302 L306 L308 L319 | L304 L320 L329 L332 | L338 L344 L347 L361 | L339 L351 L354 L355 | L340 L350 L352 L358 | L341 L345 L346 L357 | L363 L380 L386 L401 | L364 L373 L379 L402 | L365 L368 L375 L398 | L366 L372 L387 L394 | L367 L383 L391 L396 | L369 L376 L392 L400 | L370 L371 L382 L399 | L374 L378 L388 L395 | L377 L381 L385 L393 | L384 L389 L397 L403 | L390 L507 L515 L525 | L404 L414 L415 L424 | L405 L418 L426 L428 | L406 L410 L422 L432 | L407 L419 L423 L429 | L408 L446 L448 L449 | L409 L416 L425 L442 | L411 L421 L431 L433 | L412 L430 L434 L445 | L413 L417 L420 L427 | L435 L440 L443 L447 | L438 L441 A24 A25 | A26 A33 L457 L465 | L450 A30 L460 A43 | A28 L451 A29 L458 | L452 L480 A48 A49 | A31 L454 A36 L462 | A35 L464 A50 L500 | L469 L482 A52 A58 | L470 A42 L484 A47 | L474 A39 A45 L486 | L476 A46 L487 A54 | A44 L483 L498 A56 | L489 L491 L496 L550 | L490 L493 L504 L505 | L492 L502 L503 L514 | L494 L497 L520 L535 | L499 L501 L519 L542 | L506 L509 L543 L547 | L508 L511 L516 L527 | L510 L517 L540 L554 | L512 L523 L524 L545 | L513 L518 L522 L541 | L521 L526 L548 L551 | L528 L532 L539 L549 | L529 L531 L533 L544 | L530 L538 L552 L553 | L534 L536 L537 L546 makes body 1 in component "PCB"
extrude "Extrude2" add sketch "DXF import" along normal blind 2.2 contours L131 L136 L140 L164 L167 L169 | L142 L143 L151 L155 L159 L160 L164 L166 L171 L174 | L135 L152 L166 L192 L194 L207 | L144 L148 L173 L174 L190 L212 | L187 L188 L201 L204 L219 L250 | L181 L202 L215 L218 L251 L253 | L184 L185 L197 L201 L203 L206 L214 L218 L223 L231 | L197 L198 L205 L216 L236 L256 | L230 L257 L273 L275 L284 L285 | L227 L233 L239 L241 L252 L257 L262 L278 L281 L286 | L226 L242 L244 L252 L267 L282 | L221 L229 L241 L245 L259 L269 | L258 L260 L264 L266 L268 L299 L314 L316 L321 L336 | L280 L291 L316 L317 L330 L335 | L272 L296 L305 L328 L331 L336 | L268 L279 L292 L295 L313 L325 bodies 1 in component "PCB"
extrude "Extrude3" add sketch "DXF import" along normal blind 8.8 contours L131 L147 L163 L170 L177 L207 | L147 L155 L167 L189 | L143 L177 L189 L194 | L132 L136 L141 L190 L193 L195 | L140 L151 L154 L193 | L148 L154 L160 L195 | L146 L150 L165 L179 L191 L192 L209 L212 | L152 L171 L178 L191 | L159 L178 L196 L209 | L142 L144 L179 L196 | L180 L181 L183 L186 L199 L208 L217 L219 | L188 L199 L214 L237 | L187 L225 L228 L235 L247 L256 | L183 L185 L211 L215 | L202 L205 L210 L213 L232 L240 | L184 L208 L211 L237 | L200 L204 L231 L247 | L182 L206 L210 L253 | L198 L200 L203 L225 | L182 L213 L223 L236 | L220 L224 L229 L238 L246 L273 L277 L289 | L222 L226 L234 L243 L248 L285 | L224 L255 L284 L286 | L234 L275 L278 L293 | L246 L254 L255 L281 | L227 L244 L248 L293 | L238 L239 L245 L254 | L242 L269 L270 L274 L276 L298 | L233 L249 L267 L270 | L221 L249 L262 L276 | L258 L271 L294 L317 | L271 L297 L315 L321 | L283 L287 L288 L294 L305 L315 L322 L330 | L266 L296 L297 L322 | L299 L333 L334 L335 | L261 L292 L314 L334 | L261 L263 L265 L291 L313 L333 | L260 L272 L303 L323 | L264 L295 L310 L323 | L290 L303 L310 L311 L325 L331 bodies 1 in component "PCB"
extrude "Extrude4" add sketch "DXF import" along normal blind 8.5 contours L363 L380 L386 L401 | L364 L373 L379 L402 | L365 L368 L375 L398 | L366 L372 L387 L394 | L367 L383 L391 L396 | L369 L376 L392 L400 | L370 L371 L382 L399 | L374 L378 L388 L395 | L377 L381 L385 L393 | L384 L389 L397 L403 | L390 L507 L515 L525 | L404 L414 L415 L424 | L405 L418 L426 L428 | L406 L410 L422 L432 | L407 L419 L423 L429 | L408 L446 L448 L449 | L409 L416 L425 L442 | L411 L421 L431 L433 | L412 L430 L434 L445 | L413 L417 L420 L427 | L435 L440 L443 L447 | L489 L491 L496 L550 | L490 L493 L504 L505 | L492 L502 L503 L514 | L494 L497 L520 L535 | L499 L501 L519 L542 | L506 L509 L543 L547 | L508 L511 L516 L527 | L510 L517 L540 L554 | L512 L523 L524 L545 | L513 L518 L522 L541 | L521 L526 L548 L551 | L528 L532 L539 L549 | L529 L531 L533 L544 | L530 L538 L552 L553 | L534 L536 L537 L546 bodies 1 in component "PCB"
chamfer "Chamfer1" distance 0.5 angle 45 28 edges at (2.6987, 18.5738, 8.8) (6.8262, 27.4638, 8.8) (9.3663, 24.0507, 8.8) (9.3663, 13.0968, 8.8) (6.8262, 9.6837, 8.8) (2.7781, 27.4638, 8.8) (2.7781, 9.6837, 8.8) (48.7937, 9.65, 8.8) (51.3338, 12.19, 8.8) (44.7456, 9.65, 8.8) (44.6662, 16, 8.8) (44.7456, 22.35, 8.8) (48.7938, 22.35, 8.8) (51.3338, 19.81, 8.8) (44.7456, 26.11, 8.8) (48.7937, 26.11, 8.8) (44.6662, 35, 8.8) (51.3338, 29.5231, 8.8) (51.3338, 40.4769, 8.8) (48.7938, 43.89, 8.8) (44.7456, 43.89, 8.8) (32.4769, 53.3338, 8.8) (35.89, 50.7937, 8.8) (35.89, 46.7456, 8.8) (27, 46.6662, 8.8) (18.11, 46.7456, 8.8) (18.11, 50.7938, 8.8) (21.5231, 53.3338, 8.8) on bodies 1 in component "PCB"
extrude "Extrude5" add sketch "DXF import" against normal blind 0.5 from surface at -1.6 contours L3 L120 L126 L468 L475 A53 | L3 L120 L126 L157 | L3 L51 L99 L472 A51 L495 | L3 L51 L99 L157 | L3 L38 L39 L157 | L3 L38 L39 L437 A23 L444 | L3 L90 L119 A38 L473 L479 | L3 L90 L119 L157 | L3 L53 L54 L157 | L3 L53 L54 L436 L453 A34 | L3 L84 L102 L481 L485 A57 | L3 L84 L102 L157 | L3 L72 L82 L157 | L3 L72 L82 A37 L478 L488 | L3 L83 L87 L471 L477 A55 | L3 L83 L87 L157 | L3 L59 L62 L157 | L3 L59 L62 L439 L461 A41 | L3 L86 L88 A27 L455 L459 | L3 L86 L88 L157 | L3 L43 L77 L157 | L3 L43 L77 A32 L456 L467 | L3 L66 L68 L463 L466 A40 | L3 L66 L68 L157 bodies 1 in component "PCB"
extrude "Extrude6" add sketch "DXF import" against normal blind 8.8 from surface at 4 contours L3 L101 L125 L130 L157 | L91 L94 L95 L96 L97 L100 L108 L109 L113 L114 L117 L123 L124 L133 L134 L137 L138 L157 L158 L161 L175 L176 L362 | L3 L56 L58 L60 L157 | L3 L28 L41 L42 L157 | L3 L85 L92 L118 L157 | L3 L31 L34 L40 L157 | L3 L61 L64 L127 L157 | L3 L52 L73 L74 L157 | L3 L65 L89 L98 L157 | L3 L63 L70 L76 L157 | L3 L50 L57 L93 L157 | L3 L71 L78 L81 L157 | L3 L69 L75 L79 L157 | L3 L55 L67 L80 L157 bodies 1 in component "PCB"
ref_plane "WorkPlane1" through (0, 0, -4.4) normal (0, 0, 1) x (1, 0, 0) in component "diag_up_bottom"
sketch "bottom_shell" plane through (0, 0, -4.4) normal (0, 0, 1) x (1, 0, 0) in component "diag_up_bottom"
  circle A0 centre (49, 51) radius 1.5875 construction
  line L0 (1, 0) -> (52, 0) construction
  line L1 (0, 1) -> (0, 54) construction
  line L2 (53, 1) -> (53, 54) construction
  circle A1 centre (4, 51) radius 1.5875 construction
  line L3 (52, 55) -> (1, 55) construction
  line L4 (-7.5, 57.5) -> (60.5, 57.5)
  line L5 (63.5, 54.5) -> (63.5, 3)
  line L6 (60.5, 0) -> (-7.5, 0)
  line L7 (-10.5, 3) -> (-10.5, 54.5)
  arc A2 (-7.5, 57.5) -> (-10.5, 54.5) centre (-7.5, 54.5) ccw
  arc A3 (63.5, 54.5) -> (60.5, 57.5) centre (60.5, 54.5) ccw
  arc A4 (60.5, 0) -> (63.5, 3) centre (60.5, 3) ccw
  arc A5 (-10.5, 3) -> (-7.5, 0) centre (-7.5, 3) ccw
  arc A6 (61.5, 54.5) -> (60.5, 55.5) centre (60.5, 54.5) ccw
  line L8 (-7.5, 55.5) -> (60.5, 55.5)
  arc A7 (-7.5, 55.5) -> (-8.5, 54.5) centre (-7.5, 54.5) ccw
  line L9 (-8.5, 3) -> (-8.5, 54.5)
  arc A8 (-8.5, 3) -> (-7.5, 2) centre (-7.5, 3) ccw
  line L10 (60.5, 2) -> (-7.5, 2)
  arc A9 (60.5, 2) -> (61.5, 3) centre (60.5, 3) ccw
  line L11 (61.5, 54.5) -> (61.5, 3)
  arc A10 (62.3, 54.5) -> (60.5, 56.3) centre (60.5, 54.5) ccw
  line L12 (-7.5, 56.3) -> (60.5, 56.3)
  arc A11 (-7.5, 56.3) -> (-9.3, 54.5) centre (-7.5, 54.5) ccw
  line L13 (-9.3, 3) -> (-9.3, 54.5)
  arc A12 (-9.3, 3) -> (-7.5, 1.2) centre (-7.5, 3) ccw
  arc A13 (60.5, 1.2) -> (62.3, 3) centre (60.5, 3) ccw
  line L14 (62.3, 54.5) -> (62.3, 3)
  circle A14 centre (49, 51) radius 1.75
  circle A15 centre (49, 51) radius 3
  circle A16 centre (49, 51) radius 4.25
  circle A17 centre (4, 51) radius 1.75
  circle A18 centre (4, 51) radius 3
  circle A19 centre (4, 51) radius 4.25
  circle A20 centre (-4.25, 12) radius 1.75
  circle A21 centre (-4.25, 12) radius 3
  circle A22 centre (-4.25, 12) radius 4
  line L15 (-0.3, 2) -> (-0.3, 0)
  line L16 (53.3, 2) -> (53.3, 0)
  circle A23 centre (57.25, 12) radius 1.75
  circle A24 centre (57.25, 12) radius 3
  circle A25 centre (57.25, 12) radius 4
  line L17 (60.5, 1.2) -> (53, 1.2)
  line L18 (0, 1.2) -> (-7.5, 1.2)
  line L19 (26.5, 55) -> (26.5, 2) construction
  line L20 (-5.7027, 21) -> (58.2376, 21) construction
  line L21 (-2, 22) -> (2, 22)
  line L22 (2, 22) -> (2, 20)
  line L23 (2, 20) -> (-2, 20)
  line L24 (-2, 20) -> (-2, 22)
  line L25 (-0.3, 22) -> (-0.3, 20)
  line L26 (51, 22) -> (55, 22)
  line L27 (55, 22) -> (55, 20)
  line L28 (55, 20) -> (51, 20)
  line L29 (51, 20) -> (51, 22)
  line L30 (54, 22) -> (53.3, 22)
  line L31 (53.3, 22) -> (53.3, 20)
  line L32 (53.3, 20) -> (54, 20)
  point P0 (49, 51)
  point P1 (49, 51)
  dimension "d47" = 57.5
  dimension "d48" = 3
  dimension "d49" = 10.5
  dimension "d50" = 74
  dimension "d51" = 2
  dimension "d53" = 3.5
  dimension "d54" = 6
  dimension "d56" = 3.5
  dimension "d57" = 6
  dimension "d58" = 8.5
  dimension "d59" = 4.25
  dimension "d60" = 10
  dimension "d61" = 3.5
  dimension "d62" = 6
  dimension "d63" = 8
  dimension "d64" = 0.3
  dimension "d65" = 0.3
  dimension "d66" = 3.5
  dimension "d67" = 4.25
  dimension "d68" = 10
  dimension "d69" = 6
  dimension "d70" = 8
  dimension "d71" = 8.5
  dimension "d72" = 1.2
  dimension "d85" = 19
  dimension "d86" = 4
  dimension "d87" = 2
  dimension "d88" = 0.3
  dimension "d89" = 4
  dimension "d90" = 2
  dimension "d91" = 0.3
  constraint horizontal L4
  constraint vertical L5
  constraint horizontal L6
  constraint vertical L7
  constraint collinear L0 L6
  constraint tangent L4 A2
  constraint tangent L7 A2
  constraint tangent L4 A3
  constraint tangent L5 A3
  constraint equal A2 A3
  constraint tangent L5 A4
  constraint tangent L6 A4
  constraint equal A2 A4
  constraint tangent L6 A5
  constraint tangent L7 A5
  constraint equal A2 A5
  constraint coincident P0 A0.centre
  constraint concentric A14 A15
  constraint concentric A15 A16
  constraint concentric A1 A17
  constraint concentric A1 A18
  constraint concentric A17 A19
  constraint concentric A20 A21
  constraint concentric A20 A22
  constraint coincident L10 L15.start
  constraint coincident L6 L15.end
  constraint perpendicular L6 L15
  constraint coincident L10 L16.start
  constraint coincident L6 L16.end
  constraint perpendicular L6 L16
  constraint concentric A23 A24
  constraint concentric A24 A25
  constraint concentric A3 A10
  constraint parallel L4 L12
  constraint concentric A2 A11
  constraint parallel L7 L13
  constraint concentric A5 A12
  constraint parallel L6 L17
  constraint concentric A4 A13
  constraint parallel L5 L14
  constraint tangent A10 L14
  constraint tangent A13 L17
  constraint tangent A10 L12
  constraint tangent A13 L14
  constraint tangent L12 A11
  constraint tangent A11 L13
  constraint tangent A12 L17
  constraint tangent L13 A12
  constraint coincident L2 L17.end
  constraint coincident L1 L18.start
  constraint collinear L17 L18
  constraint midpoint L3 L19.start
  constraint midpoint L10 L19.end
  constraint perpendicular L2 L20
  constraint horizontal L21
  constraint vertical L22
  constraint horizontal L23
  constraint vertical L24
  constraint symmetric L20 L21 L23
  constraint symmetric L1 L22 L24
  constraint coincident L21 L25.start
  constraint coincident L23 L25.end
  constraint perpendicular L23 L25
  constraint horizontal L26
  constraint vertical L27
  constraint horizontal L28
  constraint vertical L29
  constraint horizontal L30
  constraint vertical L31
  constraint horizontal L32
  constraint coincident L28 L31.end
  constraint coincident L26 L30.start
  constraint symmetric L20 L26 L28
  constraint symmetric L2 L27 L29
  measures "d47" distance of L4 L6
  measures "d48" radius of A2
  measures "d49" distance of L1 L7
  measures "d50" distance of L5 L7
  measures "d53" diameter of A14
  measures "d54" diameter of A15
  measures "d56" diameter of A17
  measures "d57" diameter of A18
  measures "d58" diameter of A19
  measures "d59" distance of L1 A20.centre
  measures "d60" distance of L10 A20.centre
  measures "d61" diameter of A20
  measures "d62" diameter of A21
  measures "d63" diameter of A22
  measures "d64" distance of L1 L15
  measures "d65" distance of L2 L16
  measures "d66" diameter of A23
  measures "d67" distance of L2 A23.centre
  measures "d68" distance of L10 A23.centre
  measures "d69" diameter of A24
  measures "d70" diameter of A25
  measures "d71" diameter of A16
  measures "d72" distance of L7 L13
  measures "d85" distance of L10 L20
  measures "d86" distance of L22 L24
  measures "d87" distance of L21 L23
  measures "d88" distance of L1 L25
  measures "d89" distance of L27 L29
  measures "d90" distance of L26 L28
  measures "d91" distance of L2 L31
extrude "Extrude1'" add sketch "bottom_shell" against normal blind 2 separate body contours L4 L5 L6 L7 A2 A3 A4 A5 A10 L12 A11 L13 A12 A13 L14 L15 L16 L17 L18 | L6 L10 L15 L16 | A6 L8 A7 L9 A8 L10 A9 L11 A10 L12 A11 L13 A12 A13 L14 L15 L16 L17 L18 | A6 L8 A7 L9 A8 L10 A9 L11 | A16 | A19 | A22 | A25 | L21 L23 L24 L25 | L21 L22 L23 L25 | L26 L28 L29 L31 | L26 L27 L28 L30 L31 L32 makes body 2 in component "diag_up_bottom"
extrude "Extrude2'" add sketch "bottom_shell" along normal blind 1 contours L6 L10 L15 L16 bodies 2 in component "diag_up_bottom"
extrude "Extrude3'" add sketch "bottom_shell" along normal blind 9.7 contours A6 L8 A7 L9 A8 L10 A9 L11 A10 L12 A11 L13 A12 A13 L14 L15 L16 L17 L18 bodies 2 in component "diag_up_bottom"
extrude "Extrude4'" add sketch "bottom_shell" along normal blind 8.7 contours L4 L5 L6 L7 A2 A3 A4 A5 A10 L12 A11 L13 A12 A13 L14 L15 L16 L17 L18 bodies 2 in component "diag_up_bottom"
extrude "Extrude5'" add sketch "bottom_shell" along normal blind 2.8 contours A15 | A16 | A18 | A19 | L21 L22 L23 L25 | L26 L28 L29 L31 bodies 2 in component "diag_up_bottom"
extrude "Extrude6'" add sketch "bottom_shell" along normal blind 4.4 contours A21 | A22 | A24 | A25 | L21 L23 L24 L25 | L26 L27 L28 L30 L31 L32 bodies 2 in component "diag_up_bottom"
chamfer "Chamfer1'" distance 1.3 angle 45 2 edges at (0.0376, 49.4631, -1.6) (45.0376, 49.4631, -1.6) on bodies 2 in component "diag_up_bottom"
fillet "Fillet1" radius 0.5 4 edges at (-7.9793, 13.4465, -4.4) (0.0376, 52.5369, -4.4) (45.0376, 52.5369, -4.4) (53.5207, 10.5535, 0) on bodies 2 in component "diag_up_bottom"
fillet "Fillet2" radius 0.5 4 edges at (0, 20, -4.4) (2, 21, -4.4) (0, 22, -4.4) (-2, 21, -4.4) on bodies 2 in component "diag_up_bottom"
fillet "Fillet3" radius 0.5 4 edges at (51, 21, -4.4) (53, 22, -4.4) (55, 21, -4.4) (53, 20, -4.4) on bodies 2 in component "diag_up_bottom"
fillet "Fillet4" radius 0.5 1 edges at (53.5207, 13.4465, -4.4) on bodies 2 in component "diag_up_bottom"
fillet "Fillet5" radius 0.5 1 edges at (-7.9793, 10.5535, 0) on bodies 2 in component "diag_up_bottom"
ref_plane "WorkPlane1" through (0, 0, 8) normal (0, 0, 1) x (1, 0, 0) in component "diag_up_top"